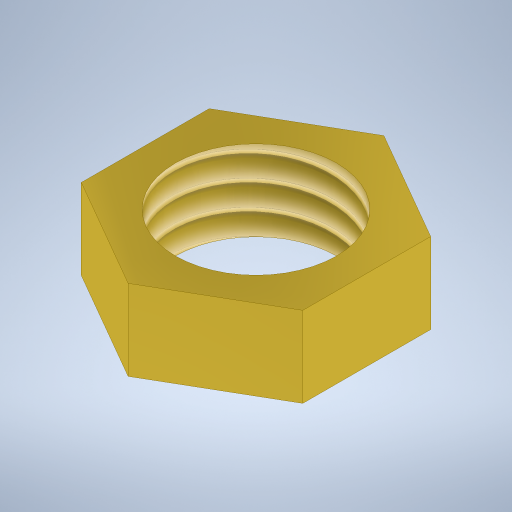
# Autodesk Inventor part: HUDSON-1-79
Saved by Autodesk Inventor 2024.2 (Build 282272000, 272)
## iProperties
Created: 2024-09-29
Part Number: HUDSON-1-79
Material: Generic
Document SubType Name: Modeling
Designer: melim
Density: 1 g/cm^3
Appearance: Metal 2400F Hot
Author: melim
Autodesk Inventor part; units mm, degrees
ref_plane "YZ Plane" through (0, 0, 0) normal (1, 0, 0) x (0, 1, 0)
ref_plane "XZ Plane" through (0, 0, 0) normal (0, 1, 0) x (-1, 0, 0)
ref_plane "XY Plane" through (0, 0, 0) normal (0, 0, 1) x (1, 0, 0)
sketch "Sketch1" plane through (0, 0, 0) normal (0, 1, 0) x (-1, 0, 0)
  line L0 (-5.5, 3.1754) -> (0, 6.3509)
  line L1 (0, 6.3509) -> (5.5, 3.1754)
  line L2 (5.5, 3.1754) -> (5.5, -3.1754)
  line L3 (5.5, -3.1754) -> (0, -6.3509)
  line L4 (0, -6.3509) -> (-5.5, -3.1754)
  line L5 (-5.5, -3.1754) -> (-5.5, 3.1754)
  line L6 (0, 7.2373) -> (0, -7.2373)
  point P0 (0, 0)
  point P1 (0, 0)
  point P2 (0, 0)
  point P3 (0, 0)
  dimension "d0" = 11
  constraints: 14 end point, 3 coincident, 1 midpoint, 1 point on line, 1 vertical, 13 other
  measures "d0" distance between parallel lines of L5 L2
extrude "Extrusion1" add sketch "Sketch1" along normal blind 4
hole "Hole1" at (0, 0, 0) direction (0, 1, 0) diameter 8 end through all
thread "Thread1" size "M8x1.25" class "6H" standard "ANSI Metric M Profile" full length
body "Solid1"
